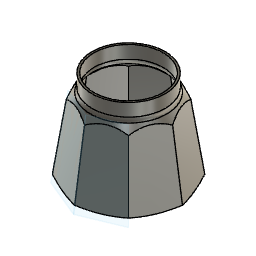
blender-01 v10 (Autodesk Fusion 360 design; units mm, degrees)
Autodesk Fusion 360 part; units mm, degrees
sketch "Sketch1" plane through (0, 0, 0) normal (0, 0, 1) x (1, 0, 0) in component "boiler"
  line L0 (38.8029, -38.8029) -> (54.8756, 0)
  line L1 (54.8756, 0) -> (38.8029, 38.8029)
  line L2 (38.8029, 38.8029) -> (0, 54.8756)
  line L3 (0, 54.8756) -> (-38.8029, 38.8029)
  line L4 (-38.8029, 38.8029) -> (-54.8756, 0)
  line L5 (-54.8756, 0) -> (-38.8029, -38.8029)
  line L6 (-38.8029, -38.8029) -> (0, -54.8756)
  line L7 (0, -54.8756) -> (38.8029, -38.8029)
  line L8 (0, 0) -> (0, -54.8756) construction
  dimension "d1" = 42
  constraint coincident L8.start origin
  constraint vertical L8
  constraint coincident L6.end L7.start
  measures "d1" distance of L0.start L6.end
extrude "Extrude1" add sketch "Sketch1" along normal blind 80 draft -8 in component "boiler"
sketch "Sketch2" plane through (-19.0257, -45.9321, 6.9872) normal (-0.378959, -0.914888, 0.139173) x (0.92388, -0.382683, 0) in component "boiler"
  line L0 (16.3429, 73.7303) -> (-16.3429, 73.7303)
  line L1 (-16.3429, 73.7303) -> (-21, -7.0559)
  line L2 (-21, -7.0559) -> (21, -7.0559)
  line L3 (21, -7.0559) -> (16.3429, 73.7303)
sketch "Sketch3" plane through (19.0257, -45.9321, 6.9872) normal (0.378959, -0.914888, 0.139173) x (0.92388, 0.382683, 0) in component "boiler"
  line L0 (16.3429, 73.7303) -> (-16.3429, 73.7303)
  line L1 (-16.3429, 73.7303) -> (-21, -7.0559)
  line L2 (-21, -7.0559) -> (21, -7.0559)
  line L3 (21, -7.0559) -> (16.3429, 73.7303)
sketch "Sketch1 (2)" plane through (0, 0, 0) normal (1, 0, 0) x (0, 1, 0)
sketch "Sketch5" plane through (0, 0, 0) normal (1, 0, 0) x (0, 1, 0) in component "boiler"
  line L0 (-65, 0) -> (-57, 9)
  line L1 (-57, 9) -> (-39, 0)
  line L2 (-39, 0) -> (-65, 0)
revolve "Revolve1" cut sketch "Sketch5" angle 360 about axis through (0, 0, 1.75) along (0, 0, 1) in component "boiler"
sketch "Sketch2 (2)" plane through (0, 0, 0) normal (0, 1, 0) x (1, 0, 0)
  line L0 (-53.7535, -7.3767) -> (-42.706, -80)
  line L1 (-30.1977, -80) -> (-42.706, -80)
  line L2 (-36.4519, -80) -> (-43.9675, -71.7075)
  constraint midpoint L1 L2.start
  constraint coincident L0 L2.end
revolve "Revolve2" cut sketch "Sketch2 (2)" angle 360 about axis through (0, 0, 1.75) along (0, 0, 1) in component "boiler"
extrude "Extrude2" add 1 faces at (9.3758, -5.1542, 80) along direction (0, 0, 1) blind 15 in component "boiler"
fillet "Fillet1" radius 6 1 edges at (33.9851, 13.1816, 80) in component "boiler"
shell "Shell1" thickness 2 removed faces 1 at (9.3758, -5.1542, 95) in component "boiler"
component "boiler" placed x (1, 0, 0) y (0, 1, 0) z (0, 0, 1) at (0, 0, 0)
